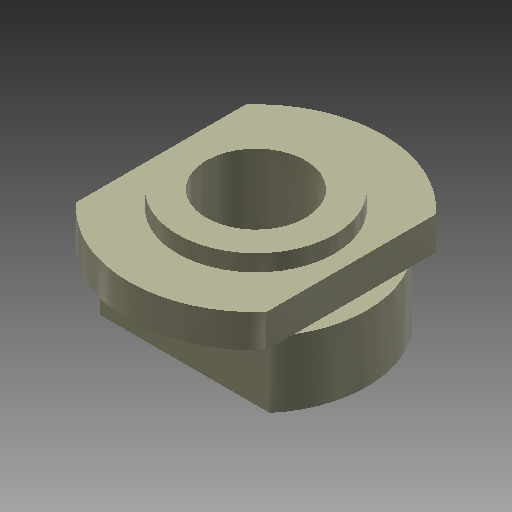
# Autodesk Inventor part: 308-08
Saved by Autodesk Inventor 2019 (Build 230136000, 136)
## iProperties
Company: Autodesk Inc.
Created: 2012-01-24
Part Number: 308-08
Material: Polypropylene
Document SubType Name: Modeling
Designer: Autodesk Inc.
Mass: 0.0694155 g
Surface Area: 1.72626 cm^2
Volume: 0.0772142 cm^3
Density: 0.899 g/cm^3
Appearance: Smooth - Ash
Author: Inventor
Autodesk Inventor part; units mm, degrees
ref_plane "YZ Plane" through (0, 0, 0) normal (1, 0, 0) x (0, 1, 0)
ref_plane "XZ Plane" through (0, 0, 0) normal (0, 1, 0) x (-1, 0, 0)
ref_plane "XY Plane" through (0, 0, 0) normal (0, 0, 1) x (1, 0, 0)
sketch "Sketch1" plane through (0, 0, 0) normal (0, 0, 1) x (1, 0, 0)
  line L0 (0, 0) -> (3.35, 0)
  line L1 (3.35, 0) -> (3.35, 2)
  line L2 (3.35, 2) -> (0, 2)
  line L3 (0, 2) -> (0, 0)
  line L4 (0, 2) -> (3.85, 2)
  line L5 (3.85, 2) -> (3.85, 3)
  line L6 (3.85, 3) -> (0, 3)
  line L7 (0, 3) -> (0, 2)
  line L8 (0, 3) -> (2.375, 3)
  line L9 (2.375, 3) -> (2.375, 3.5)
  line L10 (2.375, 3.5) -> (0, 3.5)
  line L11 (0, 3.5) -> (0, 3)
  dimension "d0" = 6.7
  dimension "d1" = 7.7
  dimension "d2" = 4.75
  dimension "d3" = 2
  dimension "d4" = 3
  dimension "d5" = 3.5
  constraints: 24 end point, 6 parallel, 3 horizontal, 3 perpendicular
  measures "d0" diameter of L1 L3
  measures "d1" diameter of L5 L3
  measures "d2" diameter of L9 L11
  measures "d3" distance of L0.end L1.end
  measures "d4" distance between parallel lines of L6 L0
  measures "d5" distance between parallel lines of L10 L0
revolve "Revolution1" add sketch "Sketch1" angle 360 about axis through (0, 3.5, 0) along (0, -1, 0)
sketch "Sketch2" plane through (0, 3, 0) normal (0, 1, 0) x (1, 0, 0)
  circle A0 centre (0, 0) radius 3.85 projected
  line L0 (-2.875, 2.5606) -> (-2.875, -2.5606)
  line L1 (2.875, 2.5606) -> (2.875, -2.5606)
  dimension "d7" = 5.75
  constraints: 4 end point, 4 point on circle, 2 parallel, 1 vertical
  measures "d7" distance between parallel lines of L1 L0
extrude "Extrusion1" cut sketch "Sketch2" against normal up to surface (1 mm away) contours A0 L1 | L0 A0
hole "Hole1" at (0, 3.5, 0) direction (0, -1, 0) diameter 3 end through all
sketch "Sketch3" plane through (0, 0, 0) normal (0, -1, 0) x (1, 0, 0)
  circle A0 centre (0, 0) radius 3.35 projected
  line L0 (4, 2.15) -> (4, 4.15)
  line L1 (4, 4.15) -> (-4, 4.15)
  line L2 (-4, 4.15) -> (-4, 2.15)
  line L3 (-4, 2.15) -> (4, 2.15)
  line L4 (4, -2.15) -> (4, -4.15)
  line L5 (4, -4.15) -> (-4, -4.15)
  line L6 (-4, -4.15) -> (-4, -2.15)
  line L7 (-4, -2.15) -> (4, -2.15)
  line L8 (0, 2.15) -> (0, -2.15) construction
  point P0 (0, 0)
  dimension "d19" = 4.3
  dimension "d20" = 2
  dimension "d21" = 8
  constraints: 18 end point, 4 parallel, 3 midpoint, 3 perpendicular, 2 equal length, 1 coincident, 1 vertical
  measures "d19" distance between parallel lines of L7 L3
  measures "d20" distance of L0.start L0.end
  measures "d21" distance of L0.end L1.end
extrude "Extrusion2" cut sketch "Sketch3" against normal up to surface (2 mm away) contours L3 A0 | A0 L3 L2 L1 L0 | L7 L4 L5 L6 A0 | A0 L7
body "Solid1"
